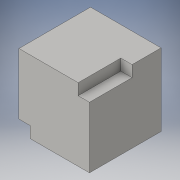
# Autodesk Inventor part: Transmission
Saved by Autodesk Inventor 2016 SP2 (Build 200236200, 236)
## iProperties
Created: 2018-01-13
Part Number: Transmission
Material: Generic
Document SubType Name: Modeling
Designer: CAD
Density: 1 g/cm^3
Appearance: Default
Author: CAD
Autodesk Inventor part; units mm, degrees
ref_plane "YZ Plane" through (0, 0, 0) normal (1, 0, 0) x (0, 1, 0)
ref_plane "XZ Plane" through (0, 0, 0) normal (0, 1, 0) x (-1, 0, 0)
ref_plane "XY Plane" through (0, 0, 0) normal (0, 0, 1) x (1, 0, 0)
sketch "Sketch1" plane through (0, 0, 0) normal (0, 0, 1) x (1, 0, 0)
  line L0 (-21.0185, 21.59) -> (21.0185, 21.59)
  line L1 (21.0185, 21.59) -> (21.0185, -21.59)
  line L2 (21.0185, -21.59) -> (-21.0185, -21.59)
  line L3 (-21.0185, -21.59) -> (-21.0185, 21.59)
  point P0 (0, 0)
  dimension "d0" = 42.037
  dimension "d1" = 43.18
  dimension "d2" = 21.59
  dimension "d3" = 21.0185
  constraints: 8 end point, 2 parallel, 1 horizontal, 1 perpendicular
  measures "d0" distance of L1.end L2.end
  measures "d1" distance of L0.end L1.end
  measures "d2" distance from line of L0 point (0, 0)
  measures "d3" distance from line of L3 point (0, 0)
extrude "Extrusion1" add sketch "Sketch1" along normal blind 42.672
sketch "Sketch2" plane through (0, 0, 42.672) normal (0, 0, 1) x (1, 0, 0)
  line L0 (21.0185, 21.59) -> (-21.0185, 21.59) projected
  line L1 (14.2875, 21.59) -> (14.2875, 14.859)
  line L2 (14.2875, 14.859) -> (21.0185, 14.859)
  line L3 (-21.0185, 21.59) -> (-21.0185, -21.59) projected
  line L4 (-21.0185, -14.859) -> (-14.2875, -14.859)
  line L5 (-14.2875, -14.859) -> (-14.2875, -21.59)
  line L6 (-21.0185, -21.59) -> (21.0185, -21.59) projected
  line L7 (21.0185, -21.59) -> (21.0185, 21.59) projected
  line L8 (14.2875, 21.59) -> (21.0185, 21.59)
  line L9 (21.0185, 21.59) -> (21.0185, 14.859)
  line L10 (-21.0185, -14.859) -> (-21.0185, -21.59)
  line L11 (-21.0185, -21.59) -> (-14.2875, -21.59)
  point P0 (0, 0)
  dimension "d6" = 6.731
  dimension "d7" = 6.731
  dimension "d8" = 6.731
  dimension "d9" = 6.731
  dimension "d10" = 0
  constraints: 16 end point, 3 point on line, 2 collinear, 2 perpendicular, 1 horizontal, 1 vertical
  measures "d6" distance of L4.end L5.end
  measures "d7" distance between parallel lines of L3 L5
  measures "d8" distance of L1.end L2.end
  measures "d9" distance of L1.start L1.end
  measures "d10" distance from line of L7 L2.end
extrude "Extrusion2" cut sketch "Sketch2" against normal blind 25.4 contours L7 L2 L1 L0 | L4 L5 L6 L3
equation "\"d2\" = 0.5 * d1"
equation "\"d3\" = 0.5 * d0"
equation "\"d6\" = d7"
equation "\"d8\" = d7"
equation "\"d9\" = d8"
body "Solid1"
